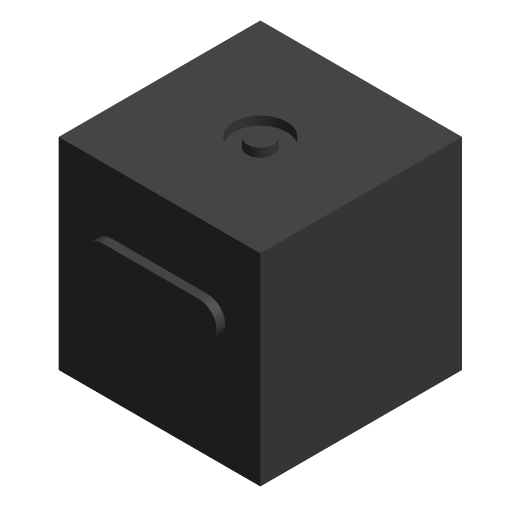
# Autodesk Inventor part: Runcam
Saved by Autodesk Inventor 2024 (Build 280153000, 153)
## iProperties
Part Number: Runcam
Material: Generic
Document SubType Name: Modeling
Designer: Jamie
Appearance: Default
Author: Jamie
Autodesk Inventor part; units mm, degrees
ref_plane "YZ Plane" through (0, 0, 0) normal (1, 0, 0) x (0, 1, 0)
ref_plane "XZ Plane" through (0, 0, 0) normal (0, 1, 0) x (-1, 0, 0)
ref_plane "XY Plane" through (0, 0, 0) normal (0, 0, 1) x (1, 0, 0)
sketch "Sketch1" plane through (0, 0, 0) normal (0, 1, 0) x (-1, 0, 0)
  line L0 (0, 0) -> (23, 0)
  line L1 (23, 0) -> (23, -23)
  line L2 (23, -23) -> (0, -23)
  line L3 (0, -23) -> (0, 0)
  dimension "d0" = 23
  dimension "d1" = 23
  constraints: 8 end point, 2 parallel, 1 horizontal, 1 perpendicular
  measures "d0" distance of L1.end L2.end
  measures "d1" distance of L0.end L1.end
extrude "Extrusion1" add sketch "Sketch1" along normal blind 23
sketch "Sketch2" plane through (0, 23, 0) normal (0, 1, 0) x (1, 0, 0)
  circle A0 centre (-11.5, 11.5) radius 1.5
  line L0 (0, 0) -> (0, 23) projected
  line L1 (-23, 0) -> (0, 0) projected
  circle A1 centre (-11.5, 11.5) radius 3
  dimension "d4" = 3
  dimension "d5" = 11.5
  dimension "d6" = 11.5
  dimension "d7" = 6
  constraints: 2 centre point, 1 coincident
  measures "d4" diameter of A0
  measures "d5" distance from line of L0 A0.centre
  measures "d6" distance from line of L1 A0.centre
  measures "d7" diameter of A1
extrude "Extrusion2" cut sketch "Sketch2" against normal blind 1
sketch "Sketch3" plane through (-23, 0, 0) normal (0, 0, 1) x (1, 0, 0)
  line L0 (6, 16) -> (19, 16)
  line L1 (17, 12) -> (6, 12)
  line L2 (0, 0) -> (0, 23) projected
  line L3 (23, 0) -> (23, 23) projected
  line L4 (0, 23) -> (23, 23) projected
  arc A0 (6, 16) -> (6, 12) centre (6, 14) ccw
  arc A1 (17, 12) -> (17, 16) centre (17, 14) ccw
  point P0 (4, 14)
  dimension "d13" = 7
  dimension "d16" = 4
  dimension "d17" = 6
  dimension "d18" = 6
  constraints: 5 point on circle, 4 end point, 4 tangent, 2 centre point, 1 horizontal, 1 parallel, 1 point on line
  measures "d13" distance between parallel lines of L4 L0
  measures "d16" distance between parallel lines of L0 L1
  measures "d17" distance from line of L2 A0.centre
  measures "d18" distance from line of L3 A1.centre
extrude "Extrusion3" add sketch "Sketch3" along normal blind 1
body "Solid1"
